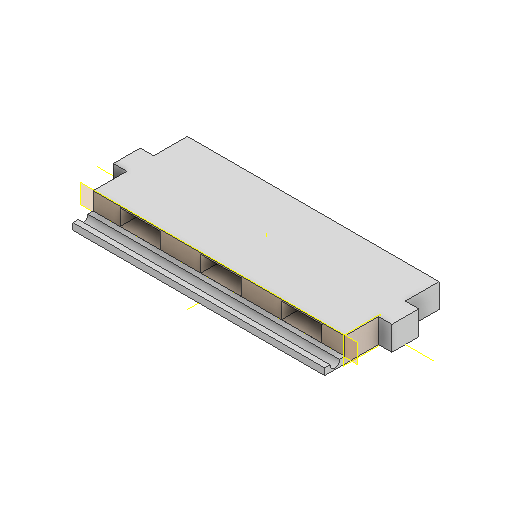
# Autodesk Inventor part: 분류대_ROW
Saved by Autodesk Inventor 2027 (Build 310192000, 192)
## iProperties
Created: 2026-09-16
Part Number: 분류대_ROW
Material: 일반
Document SubType Name: Modeling
Designer: User
Density: 1 g/cm^3
Appearance: 기본값
Author: User
Autodesk Inventor part; units mm, degrees
ref_plane "YZ 평면_우측면도" through (0, 0, 0) normal (1, 0, 0) x (0, 1, 0)
ref_plane "XZ 평면_평면도" through (0, 0, 0) normal (0, 1, 0) x (-1, 0, 0)
ref_plane "XY 평면_정면도" through (0, 0, 0) normal (0, 0, 1) x (1, 0, 0)
sketch "스케치4" plane through (0, 0, 0) normal (0, 1, 0) x (-1, 0, 0)
  line L0 (-93.5, 35) -> (93.5, 35)
  line L1 (93.5, -35) -> (-93.5, -35)
  line L2 (-93.5, 35) -> (93.5, -35) construction
  line L3 (93.5, 35) -> (-93.5, -35) construction
  line L4 (103.5, 10) -> (103.5, -10)
  line L5 (83.5, 10) -> (103.5, -10) construction
  line L6 (103.5, 10) -> (83.5, -10) construction
  line L7 (103.5, -10) -> (93.5, -10)
  line L8 (103.5, 10) -> (93.5, 10)
  line L9 (93.5, 35) -> (93.5, 10)
  line L10 (93.5, -10) -> (93.5, -35)
  line L11 (144.9, 0) -> (-144.9, 0) projected
  line L12 (0, -49) -> (0, 49) projected
  line L13 (-103.5, 10) -> (-103.5, -10)
  line L14 (-103.5, -10) -> (-93.5, -10)
  line L15 (-103.5, 10) -> (-93.5, 10)
  line L16 (-93.5, -35) -> (-93.5, -10)
  line L17 (-93.5, 10) -> (-93.5, 35)
  point P0 (0, 0)
  point P1 (93.5, 0)
  point P2 (98.5, 10)
  point P3 (93.5, 0)
  dimension "d14" = 187
  dimension "d15" = 70
  dimension "d20" = 20
  dimension "d21" = 10
  dimension "d22" = 25
  constraints: 32 end point, 6 parallel, 5 midpoint, 4 perpendicular, 4 symmetric about line, 2 point on line, 1 horizontal
  measures "d14" distance of L1.start L1.end
  measures "d15" distance of L0.end L1.start
  measures "d20" distance from line of point (98.5, 10) L7
  measures "d21" distance between parallel lines of L10 L4
  measures "d22" distance between parallel lines of L1 L7
extrude "돌출2" add sketch "스케치4" along normal blind 18
ref_plane "작업 평면2" through (93.5, 0, 35) normal (1, 0, 0) x (0, 0, -1)
sketch "스케치6" plane through (93.5, 0, 35) normal (1, 0, 0) x (0, 0, -1)
  line L0 (0, 0) -> (-15, 0)
  line L1 (-15, 0) -> (-15, 5)
  line L2 (0, 4.981) -> (0, 0)
  line L3 (-15, 5) -> (-11, 5)
  line L4 (-4, 4.981) -> (0, 4.981)
  line L5 (0, 0) -> (25, 0) projected
  line L6 (25, 0) -> (25, 18) projected
  line L7 (0, 18) -> (25, 18) projected
  line L8 (0, 0) -> (0, 18) projected
  line L9 (0, 0) -> (0, 18) projected
  line L10 (-7.5, 0) -> (-7.5, 1) construction
  arc A0 (-11, 5) -> (-4, 4.981) centre (-7.5012, 4.5302) ccw
  point P0 (35, 0)
  dimension "d26" = 15
  dimension "d27" = 5
  dimension "d29" = 4
  dimension "d30" = 4
  dimension "d36" = 1
  dimension "d37" = 3.5301
  constraints: 12 end point, 3 parallel, 3 point on circle, 2 perpendicular, 1 centre point, 1 horizontal, 1 midpoint, 1 vertical
  measures "d26" distance of L1.end L2.start
  measures "d27" distance of L0.end L1.end
  measures "d29" distance from line of L3.end L1
  measures "d30" distance from line of L2 L4.start
  measures "d36" distance of L10.start L10.end
  measures "d37" radius of A0
extrude "돌출3" add sketch "스케치6" against normal blind 187 contours L0 L1 L3 A0 L4 L2
ref_plane "작업 평면3" through (-93.5, 18, 35) normal (0, 0, 1) x (1, 0, 0)
sketch "스케치7" plane through (-93.5, 18, 35) normal (0, 0, 1) x (1, 0, 0)
  line L0 (187, -13) -> (187, -18) projected
  line L1 (187, -13) -> (0, -13) projected
  line L2 (0, -18) -> (0, -13) projected
  line L3 (187, -18) -> (0, -18) projected
  line L4 (-10, 0) -> (0, 0) projected
  line L5 (0, 0) -> (0, -13) construction
  line L6 (0, -18) -> (0, 0) projected
  line L7 (20, -1) -> (20, -13)
  line L8 (50, -1) -> (50, -13)
  line L9 (80, -1) -> (80, -13)
  line L10 (110, -1) -> (110, -13)
  line L11 (140, -1) -> (140, -13)
  line L12 (170, -1) -> (170, -13)
  line L13 (0, 0) -> (187, 0) projected
  line L14 (20, -1) -> (50, -1)
  line L15 (80, -1) -> (110, -1)
  line L16 (140, -1) -> (170, -1)
  point P0 (93.5, -18)
  point P1 (187, 0)
  dimension "d41" = 20
  dimension "d42" = 30
  dimension "d43" = 30
  dimension "d44" = 30
  dimension "d45" = 30
  dimension "d46" = 30
  dimension "d48" = 12
  dimension "d49" = 12
  dimension "d50" = 12
  constraints: 20 end point, 6 parallel, 3 horizontal, 1 collinear, 1 other
  measures "d41" distance between parallel lines of L5 L7
  measures "d42" distance between parallel lines of L7 L8
  measures "d43" distance between parallel lines of L8 L9
  measures "d44" distance between parallel lines of L9 L10
  measures "d45" distance between parallel lines of L10 L11
  measures "d46" distance between parallel lines of L11 L12
  measures "d48" distance between parallel lines of L1 L14
  measures "d49" distance between parallel lines of L1 L15
  measures "d50" distance between parallel lines of L1 L16
extrude "돌출4" cut sketch "스케치7" against normal blind 50 contours L1 L11 L16 L12 | L1 L9 L15 L10 | L7 L14 L8 L1
